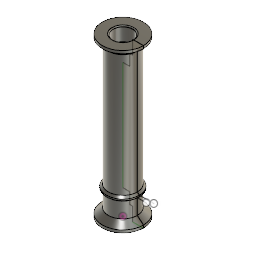
X1_Filament_Spool (Autodesk Fusion 360 design; units mm, degrees)
Autodesk Fusion 360 part; units mm, degrees
note: some values were not read from the file. Set by a fixed rule: which sketch regions a step uses.
sketch "Sketch1" plane through (0, 0, 0) normal (0, 1, 0) x (1, 0, 0)
  line L0 (0, -97) -> (5, -97)
  line L1 (0, -18) -> (5, -18)
  line L2 (5, -18) -> (5, -10)
  line L3 (7.07, -10) -> (5, -10)
  line L4 (0, -97) -> (0, -18)
  line L5 (10.5, -17) -> (12.0321, -18.2856)
  line L6 (10.5, -17) -> (16.9592, -17) construction
  line L7 (12.0321, -18.2856) -> (12.0321, -19.2856)
  line L8 (12.0321, -19.2856) -> (10.5, -20.5712)
  line L9 (12.0321, -19.2856) -> (22.4715, -19.2856) construction
  line L10 (10.5, -109.2241) -> (10.5, -20.5712)
  line L11 (15, 0) -> (7.15, 0)
  line L12 (7.07, -10) -> (7.15, 0)
  line L13 (15, 0) -> (15, -2)
  line L14 (15, -2) -> (10.5, -5.7759)
  line L15 (7.15, -115) -> (15, -115)
  line L16 (15, -115) -> (15, -113)
  line L17 (15, -113) -> (10.5, -109.2241)
  line L18 (5, -97) -> (5, -105)
  line L19 (5, -105) -> (7.07, -105)
  line L20 (7.15, -115) -> (7.07, -105)
  line L21 (10.5, -17) -> (10.5, -5.7759)
  dimension "d14" = 5
  dimension "d17" = 5
  dimension "d18" = 8
  dimension "d43" = 7.15
  dimension "d44" = 10
  dimension "d46" = 2
  dimension "d48" = 7.15
  dimension "d50" = 2
  dimension "d56" = 8
  dimension "d58" = 10
  dimension "d59" = 2
  dimension "d63" = 10.5
  dimension "d74" = 10.5
  dimension "d83" = 50
  dimension "d84" = 50
  dimension "d85" = 50
  dimension "d86" = 115
  dimension "d88" = 17
  dimension "d92" = 50
  dimension "d93" = 15
  dimension "d94" = 7.07
  dimension "d95" = 7.07
  dimension "d96" = 15
  dimension "d97" = 1
  constraint perpendicular L1 L2
  constraint horizontal L3
  constraint perpendicular L1 L4
  constraint vertical L4
  constraint horizontal L6
  constraint vertical L7
  constraint horizontal L9
  constraint vertical L10
  constraint horizontal L11
  constraint horizontal L0
  constraint perpendicular L11 L13
  constraint horizontal L15
  constraint perpendicular L15 L16
  constraint perpendicular L0 L18
  constraint perpendicular L18 L19
  constraint vertical L21
  measures "d14" distance of L0.start L0.end
  measures "d17" distance of L1.start L1.end
  measures "d18" distance of L1.end L2.end
  measures "d43" horizontal distance of origin L11.end
  measures "d44" distance of origin L3
  measures "d46" distance of L7.end L8.end
  measures "d48" distance of L4 L15.start
  measures "d50" distance of L11.start L13.end
  measures "d56" distance of L0.end L18.end
  measures "d58" distance of L15 L19
  measures "d59" distance of L15.end L16.end
  measures "d63" distance of L4 L10
  measures "d74" distance of origin L21
  measures "d83" angle of L14 L21 L19.end
  measures "d84" angle of L5 L21 L19.end
  measures "d85" angle of L8 L10
  measures "d86" distance of L11 L15
  measures "d88" distance of L5.start L11
  measures "d92" angle of L10 L17
  measures "d93" horizontal distance of origin L15.end
  measures "d94" horizontal distance of origin L19.end
  measures "d95" horizontal distance of origin L3.start
  measures "d96" distance of origin L11.start
  measures "d97" distance of L5.end L7.end
revolve "Revolve1" add sketch "Sketch1" angle 360 about axis through (0, 0, 97) along (0, 0, -1)
fillet "Fillet1" radius 0.75 1 edges at (-6.6661, -2.5856, 0)
fillet "Fillet2" radius 0.75 1 edges at (-6.6661, -2.5856, 115)
